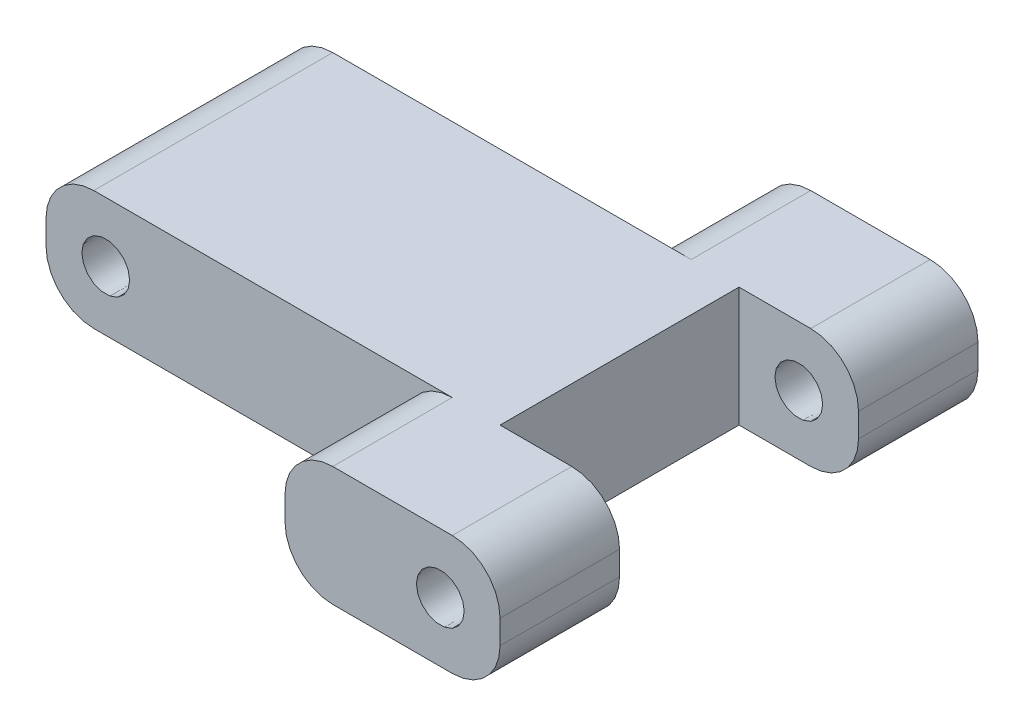
# Autodesk Inventor part: arm
Saved by Autodesk Inventor 2021 (Build 250183000, 183)
## iProperties
Created: 2020-12-29
Part Number: arm
Material: Generic
Document SubType Name: Modeling
Designer: Tomasz
Density: 1 g/cm^3
Appearance: Default
Author: Tomasz
Autodesk Inventor part; units mm, degrees
ref_plane "YZ Plane" through (0, 0, 0) normal (1, 0, 0) x (0, 1, 0)
ref_plane "XZ Plane" through (0, 0, 0) normal (0, 1, 0) x (-1, 0, 0)
ref_plane "XY Plane" through (0, 0, 0) normal (0, 0, 1) x (1, 0, 0)
sketch "arm_sketch" plane through (0, 0, 0) normal (0, 1, 0) x (-1, 0, 0)
  line L0 (0, -40) -> (-28, -40) construction
  line L1 (-28, -40) -> (-28, 0) construction
  line L2 (-28, 0) -> (0, 0) construction
  line L3 (0, 0) -> (0, -40) construction
  line L4 (0, -30) -> (-28, -30) construction
  line L5 (-28, -30) -> (-28, -10)
  line L6 (-28, -10) -> (0, -10) construction
  line L7 (0, -10) -> (0, -30) construction
  line L8 (-28, -40) -> (-38, -40)
  line L9 (-38, -40) -> (-38, -30)
  line L10 (-38, -30) -> (-28, -30)
  line L11 (-28, -30) -> (-28, -40) construction
  line L12 (0, -20) -> (-28, -20) construction
  line L13 (-14, -40) -> (-14, 0) construction
  line L14 (-28, 0) -> (-38, 0)
  line L15 (-38, 0) -> (-38, -10)
  line L16 (-38, -10) -> (-28, -10)
  line L17 (-28, -10) -> (-28, 0) construction
  line L18 (0, -40) -> (10, -40) construction
  line L19 (10, -40) -> (10, -30) construction
  line L20 (10, -30) -> (0, -30)
  line L21 (0, -30) -> (0, -40) construction
  line L22 (0, -10) -> (0, 0) construction
  line L23 (0, 0) -> (10, 0) construction
  line L24 (10, 0) -> (10, -10) construction
  line L25 (10, -10) -> (0, -10)
  line L26 (10, -30) -> (10, -10)
  line L27 (0, -10) -> (-20, -10)
  line L28 (-20, -10) -> (-20, 0)
  line L29 (0, -30) -> (-20, -30)
  line L30 (-20, -30) -> (-20, -40)
  line L31 (-20, -40) -> (-28, -40)
  line L32 (-20, 0) -> (-28, 0)
  point P0 (0, -10)
  point P1 (0, -10)
  dimension "d0" = 28
  dimension "d1" = 40
  dimension "d2" = 20
  dimension "d3" = 10
  dimension "d4" = 10
  dimension "d63" = 8
  dimension "d64" = 8
  constraints: 66 end point, 13 symmetric about line, 6 parallel, 6 point on line, 5 perpendicular, 4 midpoint, 3 horizontal, 2 coincident, 2 collinear, 1 vertical
  measures "d0" distance of L1.end L2.end
  measures "d1" distance of L0.end L1.end
  measures "d2" distance between parallel lines of L6 L4
  measures "d3" distance between parallel lines of L6 L2
  measures "d4" distance of L9.end L10.end
  measures "d63" distance between parallel lines of L1 L28
  measures "d64" distance between parallel lines of L1 L30
extrude "arm" add sketch "arm_sketch" along normal blind 10
sketch "Sketch5" plane through (20, 0, 0) normal (0, 0, 1) x (1, 0, 0)
  line L0 (18, 0) -> (18, 10) construction
  line L1 (18, 10) -> (8, 10) construction
  line L2 (-30, 0) -> (-30, 10) construction
  circle A0 centre (13, 5) radius 2
  circle A1 centre (-25, 5) radius 2
  dimension "d66" = 10
  dimension "d67" = 10
  dimension "d68" = 4
  dimension "d69" = 4
  dimension "d70" = 5
  dimension "d71" = 5
  dimension "d72" = 5
  dimension "d73" = 5
  constraints: 2 centre point
  measures "d66" distance of L0.start L0.end
  measures "d67" distance of L0.end L1.end
  measures "d68" diameter of A0
  measures "d69" diameter of A1
  measures "d70" distance from line of L2 A1.centre
  measures "d71" distance from line of A0.centre L0
  measures "d72" horizontal distance of L0.end A0.centre
  measures "d73" horizontal distance of L2.end A1.centre
extrude "rod_hole" cut sketch "Sketch5" against normal through all
fillet "rot_round" radius 4 10 edges at (-10, 10, -20) (-10, 0, -20) (38, 10, -35) (38, 0, -35) (38, 10, -5) (38, 0, -5) (20, 10, -5) (20, 0, -5) (20, 0, -35) (20, 10, -35)
equation "\"d3\" = 0.5 * d1 - 0.5 * d2"
equation "\"d64\" = d63"
equation "\"d68\" = arm_rod_diam"
equation "\"d69\" = arm_rod_diam"
equation "\"d70\" = d71"
equation "\"d71\" = 0.5 * d67"
equation "\"d72\" = 0.5 * d66"
equation "\"d73\" = d72"
equation "\"d76\" = arm_rod_diam"
equation "\"arm_rod_diam\" = 4"
equation "\"hole\" = 2.2"
body "Solid1"
